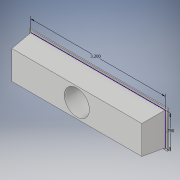
# Autodesk Inventor part: doorlatchkeeperopener
Saved by Autodesk Inventor 2019 (Build 230136000, 136)
## iProperties
Created: 2018-12-08
Part Number: doorlatchkeeperopener
Material: Generic
Document SubType Name: Modeling
Designer: User
Density: 1 g/cm^3
Appearance: Default
Author: User
Autodesk Inventor part; units mm, degrees
ref_plane "YZ Plane" through (0, 0, 0) normal (1, 0, 0) x (0, 1, 0)
ref_plane "XZ Plane" through (0, 0, 0) normal (0, 1, 0) x (-1, 0, 0)
sketch "Sketch1" plane through (0, 0, 0) normal (0, 0, 1) x (1, 0, 0)
  line L0 (0, 0) -> (81.28, 0)
  line L1 (81.28, 0) -> (81.28, 19.812)
  line L2 (81.28, 19.812) -> (0, 19.812)
  line L3 (0, 19.812) -> (0, 0)
  dimension "d0" = 81.28
  dimension "d1" = 19.812
  constraints: 8 end point, 2 parallel, 1 horizontal, 1 perpendicular
  measures "d0" distance of L1.end L2.end
  measures "d1" distance of L0.end L1.end
extrude "Extrusion1" add sketch "Sketch1" against normal blind 0.127
ref_plane "Work Plane1" through (0, 0, 12.7) normal (0, 0, 1) x (1, 0, 0)
sketch "Sketch2" plane through (0, 0, 12.7) normal (0, 0, 1) x (1, 0, 0)
  line L0 (0, 0) -> (81.28, 0) projected
  line L1 (81.28, 0) -> (81.28, 19.812) projected
  line L2 (81.28, 19.812) -> (0, 19.812) projected
  line L3 (0, 19.812) -> (0, 0) projected
  line L4 (1.27, 18.542) -> (80.01, 18.542)
  line L5 (80.01, 18.542) -> (80.01, 1.27)
  line L6 (80.01, 1.27) -> (1.27, 1.27)
  line L7 (1.27, 1.27) -> (1.27, 18.542)
  dimension "d5" = 1.27
  constraints: 8 end point, 3 other
  measures "d5" distance between parallel lines of L2 L4
extrude "Extrusion2" add sketch "Sketch2" along normal blind 0.127 contours L4 L5 L6 L7
loft "Loft1" add section 1 edges at (40.64, 18.542, 12.827) (1.27, 9.906, 12.827) (40.64, 1.27, 12.827) (80.01, 9.906, 12.827) section 2 edges at (40.64, 0, 0) (81.28, 9.906, 0) (40.64, 19.812, 0) (0, 9.906, 0)
sketch "Sketch3" plane through (0, 0, -0.127) normal (0, 0, -1) x (-1, 0, 0)
  line L0 (0, 19.812) -> (-81.28, 19.812) projected
  line L1 (0, 0) -> (0, 19.812) projected
  line L2 (-81.28, 0) -> (0, 0) projected
  line L3 (-81.28, 19.812) -> (-81.28, 0) projected
  line L4 (-82.55, 21.082) -> (1.27, 21.082)
  line L5 (1.27, 21.082) -> (1.27, -1.27)
  line L6 (1.27, -1.27) -> (-82.55, -1.27)
  line L7 (-82.55, -1.27) -> (-82.55, 21.082)
  circle A0 centre (-40.64, 9.906) radius 7.62
  dimension "d12" = 1.27
  dimension "d15" = 15.24
  constraints: 8 end point, 1 centre point, 1 coincident, 3 other
  measures "d12" distance between parallel lines of L0 L4
  measures "d15" diameter of A0
extrude "Extrusion3" add sketch "Sketch3" along normal blind 0.635 contours L4 L5 L6 L7
hole "Hole1" at (40.64, 9.906, -0.127) direction (0, 0, 1) diameter 15.24 end through all
body "Solid1"
